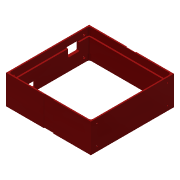
# Autodesk Inventor part: AP-02
Saved by Autodesk Inventor 2018 (Build 220112000, 112)
## iProperties
Created: 2017-11-28
Part Number: AP-02
Material: Q235
Document SubType Name: Modeling
Designer: Lars von Hebel
Mass: 200.106 g
Surface Area: 233.536 cm^2
Volume: 25.4912 cm^3
Density: 7.85 g/cm^3
Appearance: Red
RuleStatus: InUse
Author: Lars von Hebel
Autodesk Inventor part; units mm, degrees
ref_plane "YZ Plane" through (0, 0, 0) normal (1, 0, 0) x (0, 1, 0)
ref_plane "XZ Plane" through (0, 0, 0) normal (0, 1, 0) x (-1, 0, 0)
ref_plane "XY Plane" through (0, 0, 0) normal (0, 0, 1) x (1, 0, 0)
sketch "Sketch1" plane through (0, 0, 0) normal (0, 0, 1) x (1, 0, 0)
  line L0 (-45.15, -44.25) -> (45.15, -44.25)
  line L1 (45.15, -44.25) -> (45.15, 44.25)
  line L2 (45.15, 44.25) -> (-45.15, 44.25)
  line L3 (-45.15, 44.25) -> (-45.15, -44.25)
  line L4 (-45.15, -44.25) -> (45.15, 44.25) construction
  line L5 (45.15, -44.25) -> (-45.15, 44.25) construction
  line L6 (42.15, -41.25) -> (-42.15, -41.25)
  line L7 (-42.15, -41.25) -> (-42.15, 41.25)
  line L8 (-42.15, 41.25) -> (42.15, 41.25)
  line L9 (42.15, 41.25) -> (42.15, -41.25)
  line L10 (42.15, -41.25) -> (-42.15, 41.25) construction
  line L11 (-42.15, -41.25) -> (42.15, 41.25) construction
  point P0 (0, 0)
  dimension "d0" = 90.3
  dimension "d1" = 88.5
  dimension "d2" = 84.3
  dimension "d3" = 82.5
  constraints: 24 end point, 4 midpoint, 4 parallel, 2 horizontal, 2 perpendicular
  measures "d0" distance of L2.end L1.end
  measures "d1" distance of L1.end L0.end
  measures "d2" distance of L7.end L8.end
  measures "d3" distance of L6.end L7.end
extrude "Extrusion1" add sketch "Sketch1" along normal mid plane 31
sketch "Sketch2" plane through (0, 0, -15.5) normal (0, 0, -1) x (-1, 0, 0)
  line L0 (42.15, 41.25) -> (42.15, -41.25) projected
  line L1 (42.15, -41.25) -> (-42.15, -41.25) projected
  line L2 (-42.15, -41.25) -> (-42.15, 41.25) projected
  line L3 (-42.15, 41.25) -> (42.15, 41.25) projected
  line L4 (41.25, -42.85) -> (-41.25, -42.85)
  line L5 (-43.75, -40.35) -> (-43.75, 40.35)
  line L6 (-41.25, 42.85) -> (41.25, 42.85)
  line L7 (43.75, 40.35) -> (43.75, -40.35)
  line L8 (43.75, -42.85) -> (-43.75, 42.85) construction
  line L9 (-43.75, -42.85) -> (43.75, 42.85) construction
  arc A0 (-41.25, 42.85) -> (-43.75, 40.35) centre (-41.25, 40.35) ccw
  arc A1 (-43.75, -40.35) -> (-41.25, -42.85) centre (-41.25, -40.35) ccw
  arc A2 (41.25, -42.85) -> (43.75, -40.35) centre (41.25, -40.35) ccw
  arc A3 (43.75, 40.35) -> (41.25, 42.85) centre (41.25, 40.35) ccw
  point P0 (0, 0)
  dimension "d8" = 2.5
  dimension "d40" = 1.6
  dimension "d41" = 1.6
  constraints: 12 end point, 8 point on circle, 8 point on line, 8 tangent, 4 centre point, 3 equal radius, 2 midpoint, 2 parallel, 1 horizontal, 1 perpendicular
  measures "d8" radius of A0
  measures "d40" distance between parallel lines of L6 L3
  measures "d41" distance between parallel lines of L5 L2
extrude "Extrusion2" cut sketch "Sketch2" against normal blind 8
mirror "Mirror1" about plane through (0, 0, 0) normal (0, 0, 1) of "Extrusion2"
sketch "Sketch3" plane through (-45.15, -44.25, 15.5) normal (-1, 0, 0) x (0, -1, 0)
  line L0 (0, 0) -> (0, -31) projected
  line L1 (-9, -26.4) -> (-9, -20.4)
  line L2 (-10, -19.4) -> (-28, -19.4)
  line L3 (-29, -20.4) -> (-29, -26.4)
  arc A0 (-28, -19.4) -> (-29, -20.4) centre (-28, -20.4) ccw
  arc A1 (-9, -20.4) -> (-10, -19.4) centre (-10, -20.4) ccw
  line L4 (-29, -26.4) -> (-9, -26.4)
  line L5 (0, -31) -> (-88.5, -31) projected
  point P0 (-44.25, -15.5)
  dimension "d11" = 1
  dimension "d12" = 20
  dimension "d44" = 7
  dimension "d45" = 4.6
  dimension "d47" = 29
  constraints: 8 end point, 4 point on circle, 4 tangent, 2 centre point, 1 equal radius, 1 horizontal, 1 parallel, 1 vertical
  measures "d11" radius of A0
  measures "d12" distance between parallel lines of L3 L1
  measures "d44" distance between parallel lines of L2 L4
  measures "d45" distance between parallel lines of L5 L4
  measures "d47" distance between parallel lines of L0 L3
extrude "Elect" cut sketch "Sketch3" against normal blind 5
sketch "Sketch5" plane through (-45.15, -44.25, 15.5) normal (-1, 0, 0) x (0, 0, 1)
  line L0 (-31, 88.5) -> (0, 88.5) projected
  line L1 (-31, 0) -> (-31, 88.5) projected
  line L2 (-13.5, 72.7) -> (-10, 72.7)
  line L3 (-10, 72.7) -> (-10, 65.5)
  line L4 (-10, 65.5) -> (-13.5, 65.5)
  line L5 (-13.5, 65.5) -> (-13.5, 72.7)
  point P0 (-15.5, 44.25)
  point P1 (-11.75, 72.7)
  point P2 (-13.5, 69.1)
  dimension "d23" = 3.5
  dimension "d24" = 7.2
  dimension "d42" = 21
  dimension "d43" = 23
  constraints: 8 end point, 2 midpoint, 2 parallel, 1 horizontal, 1 perpendicular
  measures "d23" distance of L3.end L4.end
  measures "d24" distance of L2.end L3.end
  measures "d42" distance between parallel lines of L3 L1
  measures "d43" distance between parallel lines of L4 L0
extrude "Mini-usb" cut sketch "Sketch5" against normal blind 10
sketch "Sketch7" plane through (-45.15, -44.25, 15.5) normal (-1, 0, 0) x (0, 0, 1)
  line L0 (-13.5, 65.5) -> (-13.5, 72.7) projected
  line L1 (-10, 72.7) -> (-10, 65.5) projected
  line L2 (-10, 65.5) -> (-13.5, 65.5) projected
  line L3 (-10, 72.7) -> (-13.5, 72.7) projected
  line L4 (-10, 72.7) -> (-13.5, 65.5) construction
  line L5 (-13.5, 65.5) -> (-10, 65.5) projected
  line L6 (-10, 65.5) -> (-13.5, 72.7) construction
  line L7 (-15.25, 75.1) -> (-8.25, 75.1)
  line L8 (-7.25, 74.1) -> (-7.25, 64.1)
  line L9 (-8.25, 63.1) -> (-15.25, 63.1)
  line L10 (-16.25, 64.1) -> (-16.25, 74.1)
  line L11 (-16.25, 75.1) -> (-7.25, 63.1) construction
  line L12 (-7.25, 75.1) -> (-16.25, 63.1) construction
  arc A0 (-7.25, 74.1) -> (-8.25, 75.1) centre (-8.25, 74.1) ccw
  arc A1 (-15.25, 75.1) -> (-16.25, 74.1) centre (-15.25, 74.1) ccw
  arc A2 (-16.25, 64.1) -> (-15.25, 63.1) centre (-15.25, 64.1) ccw
  arc A3 (-8.25, 63.1) -> (-7.25, 64.1) centre (-8.25, 64.1) ccw
  point P0 (-15.5, 44.25)
  point P1 (-11.75, 69.1)
  dimension "d35" = 12
  dimension "d36" = 9
  dimension "d37" = 1
  constraints: 16 end point, 8 point on circle, 8 point on line, 8 tangent, 4 centre point, 3 equal radius, 3 midpoint, 2 parallel, 1 horizontal, 1 perpendicular
  measures "d35" distance of L12.start L11.end
  measures "d36" distance of L11.start L12.start
  measures "d37" radius of A0
extrude "USB" cut sketch "Sketch7" against normal blind 3
sketch "Sketch6" plane through (0, 0, 15.5) normal (0, 0, 1) x (1, 0, 0)
  line L0 (45.15, 44.25) -> (-45.15, 44.25) projected
  line L1 (-5, 44.25) -> (5, 44.25)
  line L2 (5, 44.25) -> (5, 43.55)
  line L3 (5, 43.55) -> (-5, 43.55)
  line L4 (-5, 43.55) -> (-5, 44.25)
  point P0 (0, 0)
  point P1 (0, 43.55)
  dimension "d31" = 10
  dimension "d32" = 0.7
  constraints: 8 end point, 2 parallel, 1 horizontal, 1 midpoint, 1 perpendicular, 1 point on line, 1 vertical alignment
  measures "d31" distance of L2.end L3.end
  measures "d32" distance of L1.end L2.end
extrude "Decoratie" cut sketch "Sketch6" against normal through all
mirror "Mirror2" about plane through (0, 0, 0) normal (0, 1, 0) of "Decoratie"
fillet "Fillet1" radius 1 4 edges at (42.15, 41.25, 0) (-42.15, 41.25, 0) (-42.15, -41.25, 0) (42.15, -41.25, 0)
sketch "Sketch8" plane through (45.15, -44.25, 15.5) normal (1, 0, 0) x (0, 0, -1)
  circle A0 centre (5, 6.75) radius 0.65
  circle A1 centre (5, 81.75) radius 0.65
  line L0 (0, 0) -> (0, 88.5) projected
  line L1 (5, 6.75) -> (5, 81.75) construction
  circle A2 centre (26, 6.75) radius 0.65
  circle A3 centre (26, 81.75) radius 0.65
  line L2 (31, 88.5) -> (31, 0) projected
  point P0 (15.5, 44.25)
  point P1 (5, 44.25)
  dimension "d49" = 1.3
  dimension "d51" = 75
  dimension "d52" = 5
  dimension "d55" = 5
  constraints: 4 centre point, 3 equal radius, 3 horizontal alignment, 2 end point, 1 midpoint, 1 vertical, 1 vertical alignment
  measures "d49" diameter of A0
  measures "d51" distance of L1.end L1.start
  measures "d52" distance from line of L0 L1.start
  measures "d55" distance from line of L2 A2.centre
extrude "Extrusion8" cut sketch "Sketch8" against normal through all
sketch "Sketch9" plane through (-43.75, -40.35, 15.5) normal (1, 0, 0) x (0, 0, -1)
  circle A0 centre (5, 2.85) radius 0.65 projected
  circle A1 centre (26, 2.85) radius 0.65 projected
  circle A2 centre (26, 77.85) radius 0.65 projected
  circle A3 centre (5, 77.85) radius 0.65 projected
  circle A4 centre (5, 77.85) radius 1.5
  circle A5 centre (5, 2.85) radius 1.5
  circle A6 centre (26, 2.85) radius 1.5
  circle A7 centre (26, 77.85) radius 1.5
  point P0 (15.5, 40.35)
  dimension "d58" = 3
  dimension "d59" = 3
  dimension "d60" = 3
  dimension "d61" = 3
  constraints: 4 centre point, 4 coincident
  measures "d58" diameter of A4
  measures "d59" diameter of A5
  measures "d60" diameter of A6
  measures "d61" diameter of A7
extrude "Extrusion9" cut sketch "Sketch9" against normal blind 0.9
mirror "Mirror3" about plane through (0, 0, 0) normal (1, 0, 0) of "Extrusion9"
body "Solid1"
